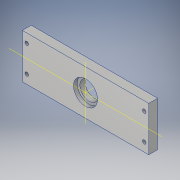
# Autodesk Inventor part: Diffbox_plate_satelite
Saved by Autodesk Inventor 2018 (Build 220112000, 112)
## iProperties
Created: 2017-10-20
Part Number: Diffbox_plate_satelite
Material: アルミニウム 6061
Document SubType Name: Modeling
Designer: 翔
Mass: 178.487 g
Surface Area: 184.864 cm^2
Volume: 66.1063 cm^3
Density: 2.7 g/cm^3
Appearance: アルミニウム - フラット
Author: 翔
Autodesk Inventor part; units mm, degrees
sketch "スケッチ3" plane through (0, 0, 0) normal (0, 1, 0) x (-1, 0, 0)
  line L0 (71, -25) -> (-71, -25)
  line L1 (-71, -25) -> (-71, 25)
  line L2 (-71, 25) -> (71, 25)
  line L3 (71, 25) -> (71, -25)
  line L4 (71, -25) -> (-71, 25) construction
  line L5 (-71, -25) -> (71, 25) construction
  point P0 (0, 0)
  dimension "d0" = 50
  dimension "d1" = 142
  constraints: 12 end point, 2 midpoint, 2 parallel, 1 horizontal, 1 perpendicular
  measures "d0" distance of L0.end L1.end
  measures "d1" distance of L1.end L2.end
extrude "押し出し1" add sketch "スケッチ3" along normal blind 10
sketch "スケッチ4" plane through (0, 0, 0) normal (0, -1, 0) x (1, 0, 0)
  circle A0 centre (0, 0) radius 13.5
  dimension "d4" = 27
  constraints: 1 centre point, 1 coincident
  measures "d4" diameter of A0
extrude "押し出し2" cut sketch "スケッチ4" against normal blind 4.1
sketch "スケッチ5" plane through (0, 4.1, 0) normal (0, -1, 0) x (1, 0, 0)
  circle A0 centre (0, 0) radius 10.5
  dimension "d7" = 21
  constraints: 1 centre point, 1 coincident
  measures "d7" diameter of A0
extrude "押し出し3" cut sketch "スケッチ5" against normal blind 10
sketch "スケッチ6" plane through (0, 0, 0) normal (0, -1, 0) x (1, 0, 0)
  circle A0 centre (-66, 15) radius 2
  line L0 (-71, 25) -> (-71, -25) projected
  line L1 (71, 25) -> (-71, 25) projected
  line L2 (-99.4, 0) -> (99.4, 0) projected
  circle A1 centre (-66, -15) radius 2
  line L3 (0, -35) -> (0, 35) projected
  circle A2 centre (66, 15) radius 2
  circle A3 centre (66, -15) radius 2
  point P0 (0, 0)
  dimension "d10" = 4
  dimension "d11" = 5
  dimension "d12" = 10
  constraints: 4 centre point, 3 symmetric about line, 3 other
  measures "d10" diameter of A0
  measures "d11" distance from line of A0.centre L0
  measures "d12" distance from line of L1 A0.centre
extrude "押し出し4" cut sketch "スケッチ6" against normal blind 10 contours A0 | A1 | A2 | A3
